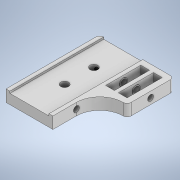
# Autodesk Inventor part: rightshortNEW1
Saved by Autodesk Inventor 2020 (Build 240168000, 168)
## iProperties
Created: 2019-12-18
Part Number: rightshortNEW1
Material: Generic
Document SubType Name: Modeling
Designer: xj82b
Density: 1 g/cm^3
Appearance: Default
Author: xj82b
Autodesk Inventor part; units mm, degrees
ref_plane "YZ Plane" through (0, 0, 0) normal (1, 0, 0) x (0, 1, 0)
ref_plane "XZ Plane" through (0, 0, 0) normal (0, 1, 0) x (-1, 0, 0)
ref_plane "XY Plane" through (0, 0, 0) normal (0, 0, 1) x (1, 0, 0)
sketch "Sketch1" plane through (0, 0, 0) normal (0, 1, 0) x (-1, 0, 0)
  line L0 (0, 0) -> (-24, 0)
  line L1 (-24, -48) -> (0, -48)
  line L2 (0, -48) -> (0, 0)
  circle A0 centre (-12, -33) radius 2
  circle A1 centre (-12, -18) radius 2
  line L3 (-24, -48) -> (-38, -48)
  line L4 (-38, -48) -> (-38, -24)
  line L5 (-38, -24) -> (-24, -24)
  line L6 (-24, -27) -> (-24, -45)
  line L7 (-24, -45) -> (-35, -45)
  line L8 (-35, -45) -> (-35, -27)
  line L9 (-35, -27) -> (-24, -27)
  line L10 (-24, -27) -> (-24, -45)
  line L11 (-24, 0) -> (-24, -24)
  line L12 (-24, -27) -> (-24, -45)
  line L13 (-28.5, -45) -> (-30.5, -45)
  line L14 (-30.5, -45) -> (-30.5, -27)
  line L15 (-30.5, -27) -> (-28.5, -27)
  line L16 (-28.5, -27) -> (-28.5, -45)
  point P0 (-12, -48)
  dimension "d0" = 24
  dimension "d1" = 48
  dimension "d2" = 4
  dimension "d3" = 4
  dimension "d4" = 15
  dimension "d5" = 30
  dimension "d6" = 14
  dimension "d7" = 24
  dimension "d8" = 3
  dimension "d9" = 3
  dimension "d10" = 3
  dimension "d11" = 48
  dimension "d12" = 11
  dimension "d27" = 18
  dimension "d28" = 4.5
  dimension "d29" = 4.5
  constraints: 34 end point, 9 parallel, 5 perpendicular, 4 horizontal, 2 centre point, 2 vertical alignment, 1 midpoint, 1 point on line
  measures "d0" distance of L1.end L1.start
  measures "d1" distance of L1.start L0.end
  measures "d2" diameter of A0
  measures "d3" diameter of A1
  measures "d4" distance from line of A0.centre L1
  measures "d5" distance from line of A1.centre L1
  measures "d6" distance of L4.end L5.end
  measures "d7" distance of L3.end L4.end
  measures "d8" distance between parallel lines of L4 L8
  measures "d9" distance between parallel lines of L5 L9
  measures "d10" distance between parallel lines of L7 L3
  measures "d11" distance between parallel lines of L0 L1
  measures "d12" distance between parallel lines of L8 L6
  measures "d27" distance of L13.end L14.end
  measures "d28" distance between parallel lines of L6 L16
  measures "d29" distance between parallel lines of L8 L14
extrude "Extrusion1" add sketch "Sketch1" along normal blind 6 contours L2 L1 L3 L4 L5 L11 L0 | L16 L7 L14 L9
sketch "Sketch2" plane through (0, 6, 0) normal (0, 1, 0) x (1, 0, 0)
  line L0 (2, 48) -> (22, 48)
  line L1 (22, 48) -> (22, 0)
  line L2 (22, 0) -> (2, 0)
  line L3 (2, 0) -> (2, 48)
  line L4 (0, 0) -> (24, 0) projected
  point P0 (12, 0)
  point P1 (12, 0)
  dimension "d15" = 20
  dimension "d16" = 48
  constraints: 8 end point, 2 midpoint, 2 parallel, 1 coincident, 1 horizontal, 1 perpendicular
  measures "d15" distance between parallel lines of L1 L3
  measures "d16" distance between parallel lines of L2 L0
extrude "Extrusion2" cut sketch "Sketch2" against normal blind 1
sketch "Sketch3" plane through (38, 0, -24) normal (1, 0, 0) x (0, 0, -1)
  circle A0 centre (12, 3) radius 1.5
  line L0 (24, 0) -> (24, 6) projected
  line L1 (0, 6) -> (24, 6) projected
  point P0 (-24, 0)
  point P1 (24, 3)
  point P2 (12, 6)
  dimension "d19" = 3
  constraints: 2 midpoint, 1 centre point, 1 horizontal alignment, 1 vertical alignment
  measures "d19" diameter of A0
extrude "Extrusion3" cut sketch "Sketch3" against normal through all
sketch "Sketch4" plane through (24, 0, 0) normal (1, 0, 0) x (0, 0, -1)
  circle A0 centre (12, 3) radius 1.5
  line L0 (0, 0) -> (0, 6) projected
  point P0 (0, 3)
  dimension "d22" = 3
  dimension "d23" = 12
  constraints: 1 centre point, 1 horizontal alignment, 1 midpoint
  measures "d22" diameter of A0
  measures "d23" distance from line of L0 A0.centre
extrude "Extrusion4" cut sketch "Sketch4" against normal through all
sketch "Sketch5" plane through (24, 0, -27) normal (1, 0, 0) x (0, 0, -1)
  circle A0 centre (9, 3) radius 1.5
  circle A1 centre (9, 3) radius 1.5 projected
  circle A2 centre (9, 3) radius 2
  point P0 (-27, 0)
  dimension "d30" = 3
  dimension "d31" = 4
  constraints: 2 centre point, 2 concentric
  measures "d30" diameter of A0
  measures "d31" diameter of A2
extrude "Extrusion5" add sketch "Sketch5" along normal blind 12
sketch "Sketch6" plane through (0, 6, 0) normal (0, 1, 0) x (1, 0, 0)
  line L0 (30.75, 42.7686) -> (34.75, 42.7686)
  line L1 (34.75, 42.7686) -> (34.75, 30.7686)
  line L2 (34.75, 30.7686) -> (30.75, 30.7686)
  line L3 (30.75, 30.7686) -> (30.75, 42.7686)
  line L4 (30.5, 27) -> (30.5, 45) projected
  line L5 (24.25, 42.1188) -> (28.25, 42.1188)
  line L6 (28.25, 42.1188) -> (28.25, 30.1188)
  line L7 (28.25, 30.1188) -> (24.25, 30.1188)
  line L8 (24.25, 30.1188) -> (24.25, 42.1188)
  line L9 (24, 27) -> (24, 45) projected
  point P0 (0, 0)
  dimension "d34" = 4
  dimension "d35" = 12
  dimension "d36" = 0.25
  dimension "d37" = 4
  dimension "d38" = 12
  dimension "d39" = 0.25
  constraints: 16 end point, 4 parallel, 2 horizontal, 2 perpendicular
  measures "d34" distance of L1.end L2.end
  measures "d35" distance of L0.end L1.end
  measures "d36" distance between parallel lines of L4 L3
  measures "d37" distance of L6.end L7.end
  measures "d38" distance of L5.end L6.end
  measures "d39" distance between parallel lines of L9 L8
extrude "Extrusion6" cut sketch "Sketch6" against normal through all
fillet "Fillet1" radius 12 1 edges at (24, 3, -24)
fillet "Fillet2" radius 2 3 edges at (38, 3, -24) (38, 3, -48) (0, 3, -48)
body "Solid1"
